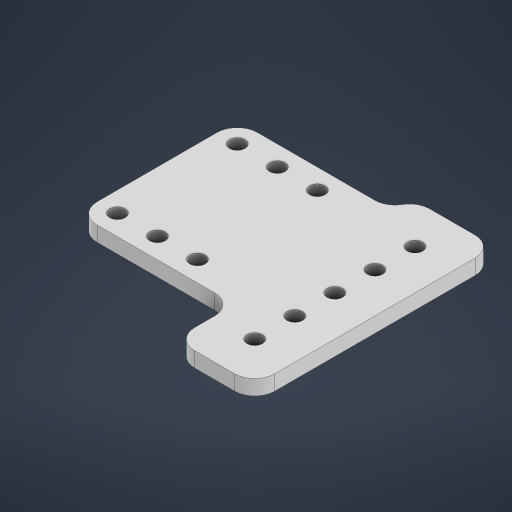
# Autodesk Inventor part: CLIM_009_BoBracket
Saved by Autodesk Inventor 2024.2 (Build 282272000, 272)
## iProperties
Created: 2024-08-08
Part Number: CLIM_009_BoBracket
Material: Generic
Document SubType Name: Modeling
Designer: Bryan
Density: 1 g/cm^3
Appearance: Default
Author: Bryan
Autodesk Inventor part; units mm, degrees
ref_plane "YZ Plane" through (0, 0, 0) normal (1, 0, 0) x (0, 1, 0)
ref_plane "XZ Plane" through (0, 0, 0) normal (0, 1, 0) x (-1, 0, 0)
ref_plane "XY Plane" through (0, 0, 0) normal (0, 0, 1) x (1, 0, 0)
sketch "Sketch1" plane through (0, 0, 0) normal (0, 1, 0) x (-1, 0, 0)
  circle A0 centre (0, 0) radius 2.4892
  line L0 (0, 0) -> (0, -25.4)
  circle A1 centre (0, -12.7) radius 2.4892
  circle A2 centre (0, -25.4) radius 2.4892
  circle A3 centre (0, -38.1) radius 2.4892
  circle A4 centre (0, -50.8) radius 2.4892
  circle A5 centre (56.3562, -12.8) radius 2.4892
  line L1 (56.3562, -12.8) -> (53.867, -12.8) construction
  circle A6 centre (43.6562, -12.8) radius 2.4892
  circle A7 centre (30.9562, -12.8) radius 2.4892
  circle A8 centre (56.3562, -50.8) radius 2.4892
  circle A9 centre (43.6562, -50.8) radius 2.4892
  circle A10 centre (30.9563, -50.8) radius 2.4892
  line L2 (-12.7, 12.7) -> (12.7, 12.7)
  line L3 (12.7, 12.7) -> (12.7, -63.5)
  line L4 (12.7, -63.5) -> (-12.7, -63.5)
  line L5 (-12.7, -63.5) -> (-12.7, 12.7)
  line L6 (62.7062, -6.35) -> (12.7, -6.35)
  line L7 (12.7, -6.35) -> (12.7, -57.15)
  line L8 (12.7, -57.15) -> (62.7062, -57.15)
  line L9 (62.7062, -57.15) -> (62.7062, -6.35)
  point P0 (41.167, -12.8)
  point P1 (28.467, -12.8)
  point P2 (53.867, -50.8)
  point P3 (41.167, -50.8)
  point P4 (28.467, -50.8)
  point P5 (12.7, -6.35)
  point P6 (0, 12.7)
  dimension "d9" = 4.9784
  dimension "d0" = 4.9784
  dimension "d1" = 25.4
  dimension "d4" = 12.7
  dimension "d12" = 12.7
  dimension "d15" = 38
  dimension "d18" = 25.4
  dimension "d19" = 76.2
  dimension "d20" = 12.7
  dimension "d22" = 18.2563
  dimension "d23" = 6.35
  dimension "d24" = 6.35
  dimension "d25" = 50.8
  dimension "d29" = 19.05
  constraints: 20 end point, 6 horizontal, 6 horizontal alignment, 6 vertical, 5 centre point, 4 parallel, 2 perpendicular, 1 coincident, 1 midpoint, 1 point on line, 1 vertical alignment, 30 other
  measures "d0" diameter of A0
  measures "d1" distance of L0.start L0.end
  measures "d4" distance of L0.start A1.centre
  measures "d12" distance of L1.start point (43.656, -12.8)
  measures "d15" distance of L1.start point (56.356, -50.8)
  measures "d18" distance of L3.end L4.end
  measures "d19" distance of L2.end L3.end
  measures "d20" distance from line of point (0, 0) L2
  measures "d22" distance from line of L3 point (30.956, -50.8)
  measures "d23" distance from line of L8 point (56.356, -50.8)
  measures "d24" distance from line of L9 point (56.356, -50.8)
  measures "d25" distance of L8.end L6.start
  measures "d29" distance between parallel lines of L2 L6
extrude "Extrusion1" add sketch "Sketch1" along normal blind 4.7625
fillet "Fillet1" radius 6.35 8 edges at (-62.7062, 2.3813, -6.35) (-12.7, 2.3813, -6.35) (-12.7, 2.3813, 12.7) (12.7, 2.3813, 12.7) (-62.7062, 2.3813, -57.15) (-12.7, 2.3813, -57.15) (-12.7, 2.3813, -63.5) (12.7, 2.3813, -63.5)
body "Solid1"
